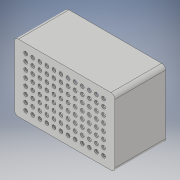
# Autodesk Inventor part: 00_Rack_Eppendorf_Tubes
Saved by Autodesk Inventor 2019.4 (Build 234330000, 330)
## iProperties
Created: 2021-04-23
Part Number: 00_Rack_Eppendorf_Tubes
Material: Generic
Document SubType Name: Modeling
Designer: diederichbenedict
Density: 1 g/cm^3
Appearance: Default
Author: diederichbenedict
Autodesk Inventor part; units mm, degrees
ref_plane "YZ Plane" through (0, 0, 0) normal (1, 0, 0) x (0, 1, 0)
ref_plane "XZ Plane" through (0, 0, 0) normal (0, 1, 0) x (-1, 0, 0)
ref_plane "XY Plane" through (0, 0, 0) normal (0, 0, 1) x (1, 0, 0)
sketch "Sketch1" plane through (0, 0, 0) normal (0, 0, 1) x (1, 0, 0)
  arc A0 (-59.9, 42.7) -> (-63.8, 38.8) centre (-59.9, 38.8) ccw projected
  arc A1 (63.8, 38.8) -> (59.9, 42.7) centre (59.9, 38.8) ccw projected
  arc A2 (59.9, -42.7) -> (63.8, -38.8) centre (59.9, -38.8) ccw projected
  arc A3 (59.9, -42.8) -> (63.9, -38.8) centre (59.9, -38.8) ccw projected
  arc A4 (-63.9, -38.8) -> (-59.9, -42.8) centre (-59.9, -38.8) ccw projected
  line L0 (-63.88, -42.74) -> (63.88, -42.74)
  line L1 (63.88, -42.74) -> (63.88, 42.74)
  line L2 (63.88, 42.74) -> (-63.88, 42.74)
  line L3 (-63.88, 42.74) -> (-63.88, -42.74)
  line L4 (-63.88, -42.74) -> (63.88, 42.74) construction
  line L5 (63.88, -42.74) -> (-63.88, 42.74) construction
  point P0 (0, 0)
  dimension "d30" = 127.76
  dimension "d31" = 85.48
  constraints: 12 end point, 2 midpoint, 2 parallel, 1 horizontal, 1 perpendicular
  measures "d30" distance of L2.end L1.end
  measures "d31" distance of L1.end L0.end
extrude "Extrusion1" add sketch "Sketch1" along normal blind 2
fillet "Fillet1" radius 5 4 edges at (63.88, 42.74, 1) (-63.88, 42.74, 1) (63.88, -42.74, 1) (-63.88, -42.74, 1)
sketch "Sketch2" plane through (0, 0, 0) normal (0, 0, -1) x (-1, 0, 0)
  line L0 (66.5944, -13.2971) -> (66.5944, -103.1184) construction
  circle A0 centre (49.5, 31.5) radius 2.375
  line L1 (63.88, 37.74) -> (63.88, -37.74) projected
  line L2 (-58.88, 42.74) -> (58.88, 42.74) projected
  dimension "d35" = 4.75
  dimension "d36" = 14.38
  dimension "d37" = 11.24
  constraints: 1 centre point
  measures "d35" diameter of A0
  measures "d36" distance from line of A0.centre L1
  measures "d37" distance from line of L2 A0.centre
extrude "Extrusion2" cut sketch "Sketch2" against normal blind 2
sketch "Sketch3" plane through (0, 0, 0) normal (0, 0, -1) x (-1, 0, 0)
  line L0 (58.795, 40.2001) -> (-58.9, 40.2001)
  arc A0 (-58.9, 40.2001) -> (-61.4, 37.7001) centre (-58.9, 37.7001) ccw
  line L1 (-61.4, 37.7001) -> (-61.4, -37.8)
  arc A1 (-61.4, -37.8) -> (-58.9, -40.3) centre (-58.9, -37.8) ccw
  line L2 (-58.9, -40.3) -> (58.795, -40.3)
  arc A2 (58.795, -40.3) -> (61.295, -37.8) centre (58.795, -37.8) ccw
  line L3 (61.295, -37.8) -> (61.295, 37.7001)
  arc A3 (61.295, 37.7001) -> (58.795, 40.2001) centre (58.795, 37.7001) ccw
  circle A4 centre (49.5, 31.5) radius 2.375 projected
  arc A5 (58.88, -42.74) -> (63.88, -37.74) centre (58.88, -37.74) ccw projected
  line L4 (63.88, 37.74) -> (63.88, -37.74) projected
  arc A6 (63.88, 37.74) -> (58.88, 42.74) centre (58.88, 37.74) ccw projected
  line L5 (-58.88, 42.74) -> (58.88, 42.74) projected
  arc A7 (-58.88, 42.74) -> (-63.88, 37.74) centre (-58.88, 37.74) ccw projected
  line L6 (-63.88, -37.74) -> (-63.88, 37.74) projected
  arc A8 (-63.88, -37.74) -> (-58.88, -42.74) centre (-58.88, -37.74) ccw projected
  line L7 (58.88, -42.74) -> (-58.88, -42.74) projected
  point P0 (0, 0)
  constraints: 8 end point, 8 point on circle, 4 centre point
extrude "Extrusion3" add sketch "Sketch3" along normal blind 62.49 contours L7 A8 L6 A7 L5 A6 L4 A5
pattern_linear "Rectangular Pattern1" count 12 spacing 9 along (1, 0, 0) count 8 spacing 9 along (0, -1, 0) of "Extrusion2"
body "Solid1"
